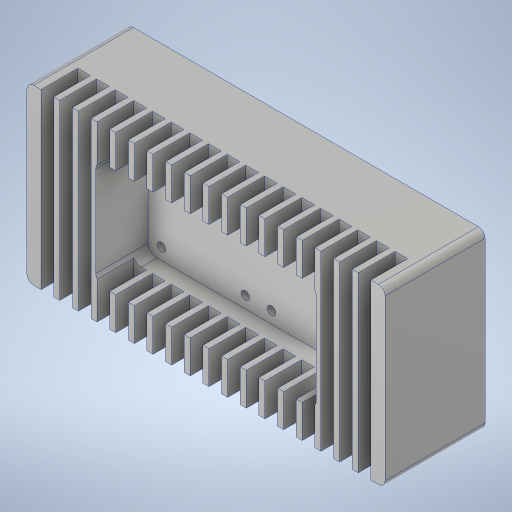
# Autodesk Inventor part: Heat sink
Saved by Autodesk Inventor 2023.4 (Build 274418000, 418)
## iProperties
Created: 2025-01-05
Part Number: Heat sink
Material: Aluminum 6061
Document SubType Name: Modeling
Designer: jmcintyr
Density: 2.7 g/cm^3
Appearance: Aluminum - Flat
Author: jmcintyr
Autodesk Inventor part; units mm, degrees
ref_plane "YZ Plane" through (0, 0, 0) normal (1, 0, 0) x (0, 1, 0)
ref_plane "XZ Plane" through (0, 0, 0) normal (0, 1, 0) x (-1, 0, 0)
ref_plane "XY Plane" through (0, 0, 0) normal (0, 0, 1) x (1, 0, 0)
sketch "Sketch1" plane through (0, 0, 0) normal (0, 0, 1) x (1, 0, 0)
  line L0 (0, 0) -> (136.525, 0)
  line L1 (136.525, 0) -> (136.525, 66.04)
  line L2 (136.525, 66.04) -> (0, 66.04)
  line L3 (0, 66.04) -> (0, 0)
  dimension "d0" = 136.525
  dimension "d1" = 66.04
  constraints: 8 end point, 2 parallel, 1 horizontal, 1 perpendicular
  measures "d0" distance of L2.end L1.end
  measures "d1" distance of L1.end L0.end
extrude "Extrusion1" add sketch "Sketch1" against normal blind 38.1
sketch "Sketch2" plane through (0, 0, 0) normal (0, 0, 1) x (1, 0, 0)
  line L0 (26.2625, 53.52) -> (110.2625, 53.52)
  line L1 (110.2625, 53.52) -> (110.2625, 12.52)
  line L2 (110.2625, 12.52) -> (26.2625, 12.52)
  line L3 (26.2625, 12.52) -> (26.2625, 53.52)
  line L4 (26.2625, 53.52) -> (110.2625, 12.52) construction
  line L5 (110.2625, 53.52) -> (26.2625, 12.52) construction
  line L6 (136.525, 66.04) -> (0, 66.04) projected
  line L7 (136.525, 0) -> (136.525, 66.04) projected
  point P0 (0, 0)
  point P1 (68.2625, 33.02)
  point P2 (68.2625, 66.04)
  point P3 (136.525, 33.02)
  dimension "d4" = 84
  dimension "d5" = 41
  constraints: 12 end point, 4 midpoint, 2 parallel, 1 horizontal, 1 horizontal alignment, 1 perpendicular, 1 vertical alignment
  measures "d4" distance of L1.end L2.end
  measures "d5" distance of L0.end L1.end
extrude "Extrusion2" cut sketch "Sketch2" against normal blind 20
fillet "Fillet1" radius 3.302 4 edges at (26.2625, 12.52, -10) (26.2625, 53.52, -10) (110.2625, 53.52, -10) (110.2625, 12.52, -10)
sketch "Sketch4" plane through (0, 0, -20) normal (0, 0, 1) x (1, 0, 0)
  arc A0 (106.9605, 12.52) -> (110.2625, 15.822) centre (106.9605, 15.822) ccw projected
  line L0 (110.2625, 50.218) -> (110.2625, 15.822) projected
  arc A1 (110.2625, 50.218) -> (106.9605, 53.52) centre (106.9605, 50.218) ccw projected
  line L1 (29.5645, 53.52) -> (106.9605, 53.52) projected
  arc A2 (29.5645, 53.52) -> (26.2625, 50.218) centre (29.5645, 50.218) ccw projected
  line L2 (26.2625, 15.822) -> (26.2625, 50.218) projected
  arc A3 (26.2625, 15.822) -> (29.5645, 12.52) centre (29.5645, 15.822) ccw projected
  line L3 (106.9605, 12.52) -> (29.5645, 12.52) projected
  line L4 (31.2625, 49.02) -> (31.2625, 17.02) construction
  line L5 (29.5645, 53.52) -> (106.9605, 53.52) construction
  line L6 (68.2625, 53.52) -> (68.2625, 12.52) construction
  line L7 (106.9605, 12.52) -> (29.5645, 12.52) construction
  point P0 (0, 0)
  point P1 (63.2625, 49.02)
  point P2 (63.2625, 17.02)
  point P3 (105.2625, 49.02)
  point P4 (73.2625, 49.02)
  point P5 (73.2625, 17.02)
  point P6 (105.2625, 17.02)
  dimension "d42" = 32
  dimension "d43" = 32
  dimension "d44" = 32
  dimension "d45" = 32
  dimension "d46" = 5
  dimension "d47" = 41
  dimension "d48" = 4.5
  constraints: 4 end point, 4 symmetric about line, 2 midpoint, 1 horizontal alignment, 1 vertical
  measures "d42" distance of L4.start point (63.262, 49.02)
  measures "d43" distance of point (63.263, 17.02) L4.end
  measures "d44" distance of point (63.262, 49.02) point (63.263, 17.02)
  measures "d45" distance of L4.start L4.end
  measures "d46" distance from line of L2 L4.end
  measures "d47" distance between parallel lines of L3 L1
  measures "d48" distance from line of L3 L4.end
sketch "Sketch5" plane through (0, 0, 0) normal (0, 0, 1) x (1, 0, 0)
  line L0 (0, 66.04) -> (0, 0) projected
  line L1 (5.3848, 66.04) -> (5.3848, 0)
  line L2 (10.2108, 66.04) -> (10.2108, 0)
  line L3 (136.525, 66.04) -> (0, 66.04) projected
  line L4 (0, 0) -> (136.525, 0) projected
  line L5 (10.2108, 66.04) -> (5.3848, 66.04)
  line L6 (10.2108, 0) -> (5.3848, 0)
  point P0 (5.3848, 50.8)
  point P1 (5.3848, 2.54)
  point P2 (10.2108, 50.8)
  point P3 (10.2108, 2.54)
  dimension "d20" = 5.3848
  dimension "d21" = 4.826
  constraints: 8 end point, 4 point on line, 2 horizontal, 2 parallel, 6 other
  measures "d20" distance between parallel lines of L0 L1
  measures "d21" distance between parallel lines of L1 L2
extrude "Extrusion3" cut sketch "Sketch5" against normal blind 14 contours L3 L2 L4 L1
pattern_linear "Rectangular Pattern1" count 18 spacing 7.112 along (1, 0, 0) of "Extrusion3"
fillet "Fillet2" radius 2.54 4 edges at (0, 0, -19.05) (136.525, 0, -19.05) (136.525, 66.04, -19.05) (0, 66.04, -19.05)
sketch "Sketch7" plane through (0, 0, -38.1) normal (0, 0, -1) x (-1, 0, 0)
  line L0 (-124.333, 5.08) -> (-12.192, 5.08)
  line L1 (-8.89, 8.382) -> (-8.89, 57.658)
  line L2 (-12.192, 60.96) -> (-124.333, 60.96)
  line L3 (-127.635, 57.658) -> (-127.635, 8.382)
  line L4 (-133.985, 0) -> (-2.54, 0) projected
  line L5 (-2.54, 66.04) -> (-133.985, 66.04) projected
  line L6 (0, 2.54) -> (0, 63.5) projected
  line L7 (-136.525, 63.5) -> (-136.525, 2.54) projected
  arc A0 (-124.333, 60.96) -> (-127.635, 57.658) centre (-124.333, 57.658) ccw
  arc A1 (-127.635, 8.382) -> (-124.333, 5.08) centre (-124.333, 8.382) ccw
  arc A2 (-12.192, 5.08) -> (-8.89, 8.382) centre (-12.192, 8.382) ccw
  arc A3 (-8.89, 57.658) -> (-12.192, 60.96) centre (-12.192, 57.658) ccw
  point P0 (0, 0)
  dimension "d29" = 118.745
  dimension "d30" = 55.88
  dimension "d31" = 66.04
  dimension "d32" = 5.08
  dimension "d33" = 136.525
  dimension "d34" = 8.89
  dimension "d35" = 3.302
  constraints: 8 end point, 8 point on circle, 8 tangent, 4 centre point, 3 equal radius, 2 parallel, 1 horizontal, 1 perpendicular
  measures "d29" distance between parallel lines of L1 L3
  measures "d30" distance between parallel lines of L2 L0
  measures "d31" distance between parallel lines of L4 L5
  measures "d32" distance between parallel lines of L0 L4
  measures "d33" distance between parallel lines of L6 L7
  measures "d34" distance between parallel lines of L6 L1
  measures "d35" radius of A0
extrude "Extrusion4" cut sketch "Sketch7" against normal blind 7.62
hole "Hole2" at (31.2625, 49.02, -20) at (63.2625, 49.02, -20) at (31.2625, 17.02, -20) at (63.2625, 17.02, -20) at (73.2625, 49.02, -20) at (105.2625, 49.02, -20) at (105.2625, 17.02, -20) at (73.2625, 17.02, -20) direction (0, 0, -1) diameter 3.302 end through all thread size "8-32 UNC" class "2B" standard "ANSI Unified Screw Threads"
equation "\"d43\" = d42"
equation "\"d44\" = d42"
equation "\"d45\" = d42"
equation "\"d48\" = -0.5 * d44 + 0.5 * d47"
equation "\"d32\" = -0.5 * d30 + 0.5 * d31"
equation "\"d34\" = -0.5 * d29 + 0.5 * d33"
body "Solid1"
